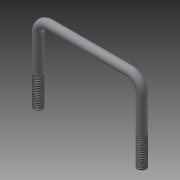
# Autodesk Inventor part: u-bolt handle
Saved by Autodesk Inventor 2015 SP1 (Build 190203100, 203)
## iProperties
Created: 2015-02-01
Part Number: u-bolt handle
Material: Generic
Document SubType Name: Modeling
Designer: Admin
Density: 1 g/cm^3
Appearance: Default
Author: Admin
Autodesk Inventor part; units mm, degrees
ref_plane "YZ Plane" through (0, 0, 0) normal (1, 0, 0) x (0, 1, 0)
ref_plane "XZ Plane" through (0, 0, 0) normal (0, 1, 0) x (-1, 0, 0)
ref_plane "XY Plane" through (0, 0, 0) normal (0, 0, 1) x (1, 0, 0)
sketch "Sketch1" plane through (0, 0, 0) normal (0, 0, 1) x (1, 0, 0)
  line L0 (0, 0) -> (0, 69.85)
  line L1 (12.7, 82.55) -> (98.425, 82.55)
  line L2 (111.125, 69.85) -> (111.125, 0)
  arc A0 (12.7, 82.55) -> (0, 69.85) centre (12.7, 69.85) ccw
  arc A1 (111.125, 69.85) -> (98.425, 82.55) centre (98.425, 69.85) ccw
  point P0 (0, 82.55)
  point P1 (111.125, 82.55)
  dimension "d0" = 82.55
  dimension "d1" = 111.125
  dimension "d2" = 82.55
  dimension "d4" = 12.7
  constraints: 6 end point, 4 point on circle, 4 point on line, 4 tangent, 2 centre point, 2 perpendicular, 1 equal radius, 1 vertical
  measures "d0" distance of L0.start point (0, 82.55)
  measures "d1" distance of point (0, 82.55) point (111.125, 82.55)
  measures "d2" distance of point (111.125, 82.55) L2.end
  measures "d4" radius of A0
sketch "Sketch2" plane through (0, 0, 0) normal (0, 1, 0) x (-1, 0, 0)
  circle A0 centre (0, 0) radius 4.7625
  dimension "d3" = 9.525
  constraints: 1 centre point, 1 coincident
  measures "d3" diameter of A0
sweep "Sweep1" add profiles "Sketch2" path "Sketch1"
thread "Thread1"
thread "Thread2"
body "Solid1"
